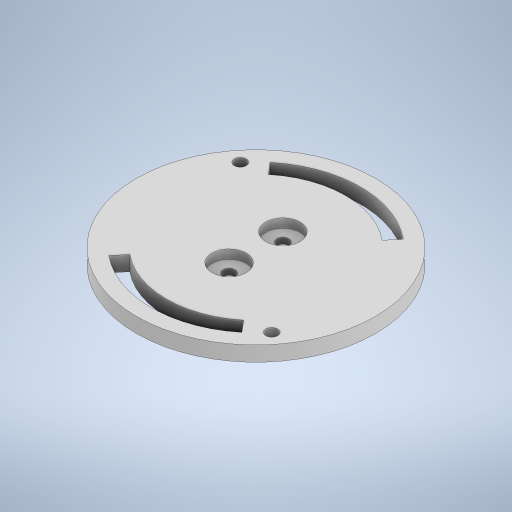
# Autodesk Inventor part: Wrist_Arm
Saved by Autodesk Inventor 2023 (Build 270158000, 158)
## iProperties
Created: 2023-02-27
Part Number: Wrist_Arm
Material: Generic
Document SubType Name: Modeling
Designer: adity
Density: 1 g/cm^3
Appearance: Default
Author: adity
Autodesk Inventor part; units mm, degrees
ref_plane "YZ Plane" through (0, 0, 0) normal (1, 0, 0) x (0, 1, 0)
ref_plane "XZ Plane" through (0, 0, 0) normal (0, 1, 0) x (-1, 0, 0)
sketch "Sketch1" plane through (0, 0, 0) normal (0, 1, 0) x (-1, 0, 0)
  circle A0 centre (0, 0) radius 40
  dimension "d0" = 80
  constraints: 1 centre point, 1 coincident
  measures "d0" diameter of A0
sketch "Sketch1 outline for Extrusion1" plane through (0, 0, 0) normal (0, 1, 0) x (-1, 0, 0)
  circle A0 centre (0, 0) radius 40
extrude "Extrusion1" add sketch "Sketch1 outline for Extrusion1" along normal blind 5
sketch "Sketch3" plane through (0, 5, 0) normal (0, 1, 0) x (1, 0, 0)
  line L0 (0, 0) -> (-5, 0)
  line L1 (0, 0) -> (5, 0)
  line L2 (0, 0) -> (0, -9)
  line L3 (0, 0) -> (0, 9)
  circle A0 centre (0, 9) radius 2
  circle A1 centre (0, -9) radius 2
  dimension "d63" = 9
  dimension "d64" = 9
  dimension "d65" = 4
  dimension "d66" = 4
  constraints: 8 end point, 3 coincident, 2 centre point, 2 horizontal, 2 vertical
  measures "d63" distance of L0.start L2.end
  measures "d64" distance of L0.start L3.end
  measures "d65" diameter of A0
  measures "d66" diameter of A1
sketch "Sketch3 outline for Extrusion3" plane through (0, 5, 0) normal (0, 1, 0) x (1, 0, 0)
  circle A0 centre (0, 9) radius 2
  circle A1 centre (0, -9) radius 2
extrude "Extrusion3" cut sketch "Sketch3 outline for Extrusion3" against normal up to surface (5 mm away)
sketch "Sketch6" plane through (0, 0, 0) normal (0, -1, 0) x (1, 0, 0)
  line L0 (0, 0) -> (-25, 0)
  line L1 (0, 0) -> (25, 0)
  circle A0 centre (25, 0) radius 10
  circle A1 centre (-25, 0) radius 10
  dimension "d18" = 25
  dimension "d19" = 25
  dimension "d20" = 20
  dimension "d21" = 20
  constraints: 4 end point, 2 centre point, 2 coincident, 2 horizontal
  measures "d18" distance of L0.start L0.end
  measures "d19" distance of L1.start L1.end
  measures "d20" diameter of A0
  measures "d21" diameter of A1
sketch "Sketch6 outline for Extrusion5" plane through (0, 0, 0) normal (0, -1, 0) x (1, 0, 0)
  circle A0 centre (25, 0) radius 10
  circle A1 centre (-25, 0) radius 10
extrude "Extrusion5" cut sketch "Sketch6 outline for Extrusion5" against normal blind 4
sketch "Sketch8" plane through (0, 0, 0) normal (0, -1, 0) x (1, 0, 0)
  circle A0 centre (0, 0) radius 40
  line L0 (0, 40) -> (0, 35)
  line L1 (0, 35) -> (0, 30)
  line L2 (0, 30) -> (0, 27)
  circle A1 centre (0, 0) radius 35
  circle A2 centre (0, 0) radius 30
  line L3 (0, 27) -> (30, 27)
  line L4 (22.271057, 27) -> (19.056987, 23.169619)
  line L5 (22.271057, 27) -> (27.271264, 27) construction
  line L6 (-40, 0) -> (40, 0)
  line L7 (22.271057, -27) -> (19.056987, -23.169619)
  line L8 (0, -40) -> (0, -30)
  point P0 (0, -35)
  dimension "d46" = 5
  dimension "d47" = 5
  dimension "d48" = 3
  dimension "d49" = 130
  constraints: 18 end point, 9 point on circle, 3 horizontal, 3 point on line, 2 centre point, 2 coincident, 2 symmetric about line, 2 vertical, 1 equal length
  measures "d46" distance of L0.start L0.end
  measures "d47" distance of L0.end L1.end
  measures "d48" distance of L1.end L2.end
  measures "d49" angle of L4 L5
sketch "Sketch8 outline for Extrusion7" plane through (0, 0, 0) normal (0, -1, 0) x (1, 0, 0)
  line L0 (0, -30) -> (0, -35)
  arc A0 (19.056987, -23.169619) -> (0, -30) centre (0, 0) cw
  line L1 (22.271057, -27) -> (19.056987, -23.169619)
  arc A1 (0, -35) -> (22.271057, -27) centre (0, 0) ccw
  arc A2 (22.271057, 27) -> (0, 35) centre (0, 0) ccw
  line L2 (19.056987, 23.169619) -> (22.271057, 27)
  arc A3 (0, 30) -> (19.056987, 23.169619) centre (0, 0) cw
  line L3 (0, 35) -> (0, 30)
extrude "Extrusion7" cut sketch "Sketch8 outline for Extrusion7" against normal up to surface (5 mm away)
ref_plane "Work Plane1" through (0, 0, 32.5) normal (1, 0, 0) x (0, 0, -1)
mirror "Mirror1" about plane through (0, 0, 32.5) normal (1, 0, 0) of "Extrusion7"
sketch "Sketch11" plane through (0, 5, 0) normal (0, 1, 0) x (1, 0, 0)
  circle A0 centre (0, -9) radius 2 projected
  circle A1 centre (0, -9) radius 5.75
  circle A2 centre (0, 9) radius 2 projected
  circle A3 centre (0, 9) radius 5.75
  point P0 (0, 0)
  dimension "d67" = 11.5
  dimension "d68" = 11.5
  constraints: 2 centre point, 2 coincident
  measures "d67" diameter of A1
  measures "d68" diameter of A3
sketch "Sketch11 outline for Extrusion10" plane through (0, 5, 0) normal (0, 1, 0) x (1, 0, 0)
  circle A0 centre (0, 9) radius 5.75
  circle A1 centre (0, 9) radius 2
  circle A2 centre (0, -9) radius 5.75
  circle A3 centre (0, -9) radius 2
extrude "Extrusion10" cut sketch "Sketch11 outline for Extrusion10" against normal blind 3
sketch "Sketch12" plane through (0, 0, 0) normal (0, -1, 0) x (1, 0, 0)
  circle A0 centre (0, 0) radius 40
  line L0 (0, -40) -> (0, -35)
  arc A1 (-22.271057, -27) -> (22.271057, -27) centre (0, 0) ccw
  arc A2 (-19.056987, -23.169619) -> (19.056987, -23.169619) centre (0, 0) ccw
  circle A3 centre (-25, 0) radius 10
  line L1 (22.271057, 27) -> (22.271057, 22)
  line L2 (22.271057, 22) -> (27.271057, 22)
  circle A4 centre (27.271057, 22) radius 2
  line L3 (-22.271057, -27) -> (-22.271057, -22)
  line L4 (-22.271057, -22) -> (-27.271057, -22)
  circle A5 centre (-27.271057, -22) radius 2
  dimension "d71" = 5
  dimension "d72" = 5
  dimension "d73" = 4
  dimension "d74" = 5
  dimension "d75" = 5
  dimension "d76" = 4
  constraints: 10 end point, 3 vertical, 2 centre point, 2 coincident, 2 perpendicular, 1 point on circle, 1 vertical alignment, 1 other
  measures "d71" distance of L1.start L1.end
  measures "d72" distance of L1.end L2.end
  measures "d73" diameter of A4
  measures "d74" distance of L3.start L3.end
  measures "d75" distance of L3.end L4.end
  measures "d76" diameter of A5
sketch "Sketch12 outline for Extrusion11" plane through (0, 0, 0) normal (0, -1, 0) x (1, 0, 0)
  circle A0 centre (-27.271057, -22) radius 2
  circle A1 centre (27.271057, 22) radius 2
extrude "Extrusion11" cut sketch "Sketch12 outline for Extrusion11" against normal up to surface (5 mm away)
body "Solid1"
